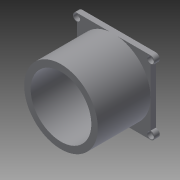
# Autodesk Inventor part: Nikon Mount
Saved by Autodesk Inventor 2013 (Build 170138000, 138)
## iProperties
Created: 2014-04-13
Part Number: Nikon Mount
Material: Generic
Document SubType Name: Modeling
Designer: spichelh
Density: 1 g/cm^3
Author: spichelh
Autodesk Inventor part; units mm, degrees
ref_plane "YZ Plane" through (0, 0, 0) normal (1, 0, 0) x (0, 1, 0)
ref_plane "XZ Plane" through (0, 0, 0) normal (0, 1, 0) x (-1, 0, 0)
ref_plane "XY Plane" through (0, 0, 0) normal (0, 0, 1) x (1, 0, 0)
sketch "Sketch1" plane through (0, 0, 0) normal (0, 0, 1) x (1, 0, 0)
  line L0 (55.88, 55.53) -> (0, 55.53)
  circle A0 centre (0, 3) radius 1.5
  arc A1 (0, 6) -> (0, 0) centre (0, 3) ccw
  circle A2 centre (0, 52.53) radius 1.5
  arc A3 (0, 55.53) -> (0, 49.53) centre (0, 52.53) ccw
  line L1 (27.94, 5) -> (27.94, 55.53) construction
  circle A4 centre (55.88, 3) radius 1.5
  arc A5 (55.88, 0) -> (55.88, 6) centre (55.88, 3) ccw
  circle A6 centre (55.88, 52.53) radius 1.5
  arc A7 (55.88, 49.53) -> (55.88, 55.53) centre (55.88, 52.53) ccw
  line L2 (55.88, 6) -> (55.88, 49.53)
  line L3 (55.88, 55.53) -> (55.88, 55.53)
  line L4 (0, 55.53) -> (0, 55.53)
  line L5 (0, 49.53) -> (0, 6)
  line L6 (52.88, 53.53) -> (3, 53.53)
  line L7 (0, 0) -> (0, 6) construction
  line L8 (55.88, 0) -> (55.88, 6) construction
  line L9 (0, 0) -> (0, 0)
  line L10 (0, 0) -> (55.88, 0)
  line L11 (55.88, 0) -> (55.88, 0)
  line L12 (50.88, 56.34) -> (5, 56.34) construction
  line L13 (3, 3) -> (52.88, 3)
  line L14 (3, 53.53) -> (3, 3)
  line L15 (52.88, 3) -> (52.88, 53.53)
  dimension "d0" = 55.88
  dimension "d2" = 3
  dimension "d3" = 6
  dimension "d4" = 3
  dimension "d5" = 6
  dimension "d6" = 49.53
  dimension "d8" = 3
  dimension "d14" = 2
  dimension "d33" = 0.81
  dimension "d78" = 3
  dimension "d79" = 3
  dimension "d214" = 0
  dimension "d215" = 3
  dimension "d216" = 0
  constraints: 32 end point, 9 parallel, 8 centre point, 8 point on circle, 5 coincident, 4 symmetric about line, 3 midpoint, 2 perpendicular, 1 collinear, 1 point on line, 4 other
  measures "d0" distance of L7.start L8.start
  measures "d2" diameter of A0
  measures "d3" diameter of A1
  measures "d4" diameter of A2
  measures "d5" diameter of A3
  measures "d6" distance of A0.centre A2.centre
  measures "d8" distance of A0.centre L7.start
  measures "d14" distance between parallel lines of L0 L6
  measures "d33" distance between parallel lines of L0 L12
  measures "d78" distance between parallel lines of L15 L2
  measures "d79" distance between parallel lines of L5 L14
  measures "d214" distance of L3.start L0.start
  measures "d215" distance between parallel lines of L10 L13
  measures "d216" distance of L9.end L7.start
extrude "Extrusion1" add sketch "Sketch1" along normal blind 4
sketch "Sketch14" plane through (0, 0, 4) normal (0, 0, 1) x (1, 0, 0)
  line L0 (3, 53.53) -> (52.88, 53.53)
  circle A0 centre (27.94, 27.765) radius 23
  line L1 (27.94, 53.53) -> (27.94, -2.5) construction
  line L2 (49.2166, 63.2696) -> (5.8766, 63.2721) construction
  line L3 (-23.2566, 6.5875) -> (78.3434, 6.5818) construction
  line L4 (-23.2534, 63.2737) -> (-23.2566, 6.5875) construction
  line L5 (78.3434, 6.5818) -> (78.3466, 63.268) construction
  line L6 (52.88, 53.53) -> (52.88, 3) projected
  line L7 (52.88, 3) -> (3, 3) projected
  line L8 (3, 3) -> (3, 53.53) projected
  line L9 (3, 3) -> (3, 53.53)
  line L10 (52.88, 53.53) -> (52.88, 3)
  line L11 (52.88, 3) -> (3, 3)
  point P0 (52.88, -2.5)
  dimension "d96" = 46
  constraints: 10 end point, 3 collinear, 1 centre point, 1 horizontal, 1 midpoint, 1 point on line
  measures "d96" diameter of A0
extrude "Extrusion14" add sketch "Sketch14" against normal blind 4
sketch "Sketch15" plane through (0, 0, 4) normal (0, 0, 1) x (1, 0, 0)
  circle A0 centre (27.94, 27.765) radius 23 projected
  line L0 (0, 49.53) -> (0, 6) projected
  circle A1 centre (27.94, 27.765) radius 27.94
  circle A2 centre (27.94, 27.765) radius 23
  dimension "d102" = 55.88
  dimension "d103" = 46
  constraints: 2 centre point, 2 coincident, 1 concentric, 1 tangent
  measures "d102" diameter of A1
  measures "d103" diameter of A0
extrude "Extrusion15" add sketch "Sketch15" along normal blind 40
sketch "Sketch17" plane through (0, 0, 0) normal (0, 0, -1) x (-1, 0, 0)
  circle A0 centre (-27.94, 27.765) radius 23 construction
  line L0 (-37.34, 35.815) -> (-18.54, 35.815)
  line L1 (-17.54, 34.815) -> (-17.54, 20.715)
  line L2 (-18.54, 19.715) -> (-37.34, 19.715)
  line L3 (-38.34, 20.715) -> (-38.34, 34.815)
  line L4 (-17.54, 35.815) -> (-38.34, 19.715) construction
  line L5 (-17.54, 19.715) -> (-38.34, 35.815) construction
  circle A1 centre (-27.94, 27.765) radius 23
  arc A2 (-37.34, 35.815) -> (-38.34, 34.815) centre (-37.34, 34.815) ccw
  arc A3 (-38.34, 20.715) -> (-37.34, 19.715) centre (-37.34, 20.715) ccw
  arc A4 (-18.54, 19.715) -> (-17.54, 20.715) centre (-18.54, 20.715) ccw
  arc A5 (-17.54, 34.815) -> (-18.54, 35.815) centre (-18.54, 34.815) ccw
  point P0 (0, 0)
  dimension "d111" = 20.8
  dimension "d112" = 16.1
  dimension "d115" = 1
  constraints: 12 end point, 8 point on circle, 8 point on line, 8 tangent, 5 centre point, 4 equal radius, 2 midpoint, 2 parallel, 1 coincident, 1 horizontal, 1 perpendicular
  measures "d111" distance of L5.start L4.end
  measures "d112" distance of L4.start L5.start
  measures "d115" radius of A2
extrude "Extrusion17" add sketch "Sketch17" against normal blind 11
sketch "Sketch18" plane through (27.94, 27.765, 11) normal (0, 0, 1) x (1, 0, 0)
  line L0 (10.4, 7.05) -> (10.4, -7.05) projected
  line L1 (9.4, -8.05) -> (-9.4, -8.05) projected
  line L2 (-10.4, -7.05) -> (-10.4, 7.05) projected
  line L3 (-9.4, 8.05) -> (9.4, 8.05) projected
  arc A0 (10.4, 7.05) -> (9.4, 8.05) centre (9.4, 7.05) ccw projected
  arc A1 (9.4, -8.05) -> (10.4, -7.05) centre (9.4, -7.05) ccw projected
  arc A2 (-10.4, -7.05) -> (-9.4, -8.05) centre (-9.4, -7.05) ccw projected
  arc A3 (-9.4, 8.05) -> (-10.4, 7.05) centre (-9.4, 7.05) ccw projected
  line L4 (9.4, 9.05) -> (-9.4, 9.05)
  arc A4 (-9.4, 9.05) -> (-11.4, 7.05) centre (-9.4, 7.05) ccw
  line L5 (-11.4, 7.05) -> (-11.4, -7.05)
  arc A5 (-11.4, -7.05) -> (-9.4, -9.05) centre (-9.4, -7.05) ccw
  line L6 (-9.4, -9.05) -> (9.4, -9.05)
  arc A6 (9.4, -9.05) -> (11.4, -7.05) centre (9.4, -7.05) ccw
  line L7 (11.4, -7.05) -> (11.4, 7.05)
  arc A7 (11.4, 7.05) -> (9.4, 9.05) centre (9.4, 7.05) ccw
  point P0 (10.4, 8.05)
  point P1 (10.4, -8.05)
  point P2 (-10.4, -8.05)
  point P3 (-10.4, 8.05)
  point P4 (-27.94, -27.765)
  dimension "d116" = 1
  constraints: 8 end point, 8 point on circle, 4 centre point, 7 other
  measures "d116" distance between parallel lines of L4 L3
extrude "Extrusion18" cut sketch "Sketch18" against normal blind 8
sketch "Sketch19" plane through (27.94, 27.765, 11) normal (0, 0, 1) x (1, 0, 0)
  arc A0 (-9.4, 9.05) -> (-11.4, 7.05) centre (-9.4, 7.05) ccw projected
  line L0 (-9.4, 9.05) -> (9.4, 9.05) projected
  arc A1 (11.4, 7.05) -> (9.4, 9.05) centre (9.4, 7.05) ccw projected
  line L1 (11.4, 7.05) -> (11.4, -7.05) projected
  arc A2 (9.4, -9.05) -> (11.4, -7.05) centre (9.4, -7.05) ccw projected
  line L2 (9.4, -9.05) -> (-9.4, -9.05) projected
  arc A3 (-11.4, -7.05) -> (-9.4, -9.05) centre (-9.4, -7.05) ccw projected
  line L3 (-11.4, -7.05) -> (-11.4, 7.05) projected
  line L4 (9.4, 10.05) -> (-9.4, 10.05)
  arc A4 (-9.4, 10.05) -> (-12.4, 7.05) centre (-9.4, 7.05) ccw
  line L5 (-12.4, 7.05) -> (-12.4, -7.05)
  arc A5 (-12.4, -7.05) -> (-9.4, -10.05) centre (-9.4, -7.05) ccw
  line L6 (-9.4, -10.05) -> (9.4, -10.05)
  arc A6 (9.4, -10.05) -> (12.4, -7.05) centre (9.4, -7.05) ccw
  line L7 (12.4, -7.05) -> (12.4, 7.05)
  arc A7 (12.4, 7.05) -> (9.4, 10.05) centre (9.4, 7.05) ccw
  point P0 (-27.94, -27.765)
  dimension "d119" = 1
  constraints: 8 end point, 8 point on circle, 4 centre point, 7 other
  measures "d119" distance between parallel lines of L0 L4
extrude "Extrusion19" cut sketch "Sketch19" against normal blind 7
sketch "Sketch20" plane through (27.94, 27.765, 11) normal (0, 0, 1) x (1, 0, 0)
  arc A0 (-9.4, 10.05) -> (-12.4, 7.05) centre (-9.4, 7.05) ccw projected
  line L0 (-9.4, 10.05) -> (9.4, 10.05) projected
  arc A1 (12.4, 7.05) -> (9.4, 10.05) centre (9.4, 7.05) ccw projected
  line L1 (12.4, 7.05) -> (12.4, -7.05) projected
  arc A2 (9.4, -10.05) -> (12.4, -7.05) centre (9.4, -7.05) ccw projected
  line L2 (9.4, -10.05) -> (-9.4, -10.05) projected
  arc A3 (-12.4, -7.05) -> (-9.4, -10.05) centre (-9.4, -7.05) ccw projected
  line L3 (-12.4, -7.05) -> (-12.4, 7.05) projected
  line L4 (9.4, 11.05) -> (-9.4, 11.05)
  arc A4 (-9.4, 11.05) -> (-13.4, 7.05) centre (-9.4, 7.05) ccw
  line L5 (-13.4, 7.05) -> (-13.4, -7.05)
  arc A5 (-13.4, -7.05) -> (-9.4, -11.05) centre (-9.4, -7.05) ccw
  line L6 (-9.4, -11.05) -> (9.4, -11.05)
  arc A6 (9.4, -11.05) -> (13.4, -7.05) centre (9.4, -7.05) ccw
  line L7 (13.4, -7.05) -> (13.4, 7.05)
  arc A7 (13.4, 7.05) -> (9.4, 11.05) centre (9.4, 7.05) ccw
  point P0 (-27.94, -27.765)
  dimension "d122" = 1
  constraints: 8 end point, 8 point on circle, 4 centre point, 7 other
  measures "d122" distance between parallel lines of L4 L0
extrude "Extrusion20" cut sketch "Sketch20" against normal blind 6
sketch "Sketch21" plane through (27.94, 27.765, 11) normal (0, 0, 1) x (1, 0, 0)
  arc A0 (-9.4, 11.05) -> (-13.4, 7.05) centre (-9.4, 7.05) ccw projected
  line L0 (-9.4, 11.05) -> (9.4, 11.05) projected
  arc A1 (13.4, 7.05) -> (9.4, 11.05) centre (9.4, 7.05) ccw projected
  line L1 (13.4, 7.05) -> (13.4, -7.05) projected
  arc A2 (9.4, -11.05) -> (13.4, -7.05) centre (9.4, -7.05) ccw projected
  line L2 (9.4, -11.05) -> (-9.4, -11.05) projected
  arc A3 (-13.4, -7.05) -> (-9.4, -11.05) centre (-9.4, -7.05) ccw projected
  line L3 (-13.4, -7.05) -> (-13.4, 7.05) projected
  line L4 (9.4, 12.05) -> (-9.4, 12.05)
  arc A4 (-9.4, 12.05) -> (-14.4, 7.05) centre (-9.4, 7.05) ccw
  line L5 (-14.4, 7.05) -> (-14.4, -7.05)
  arc A5 (-14.4, -7.05) -> (-9.4, -12.05) centre (-9.4, -7.05) ccw
  line L6 (-9.4, -12.05) -> (9.4, -12.05)
  arc A6 (9.4, -12.05) -> (14.4, -7.05) centre (9.4, -7.05) ccw
  line L7 (14.4, -7.05) -> (14.4, 7.05)
  arc A7 (14.4, 7.05) -> (9.4, 12.05) centre (9.4, 7.05) ccw
  point P0 (-27.94, -27.765)
  dimension "d125" = 1
  constraints: 8 end point, 8 point on circle, 4 centre point, 7 other
  measures "d125" distance between parallel lines of L0 L4
extrude "Extrusion21" cut sketch "Sketch21" against normal blind 5
sketch "Sketch22" plane through (27.94, 27.765, 11) normal (0, 0, 1) x (1, 0, 0)
  arc A0 (-9.4, 12.05) -> (-14.4, 7.05) centre (-9.4, 7.05) ccw projected
  line L0 (-9.4, 12.05) -> (9.4, 12.05) projected
  arc A1 (14.4, 7.05) -> (9.4, 12.05) centre (9.4, 7.05) ccw projected
  line L1 (14.4, 7.05) -> (14.4, -7.05) projected
  arc A2 (9.4, -12.05) -> (14.4, -7.05) centre (9.4, -7.05) ccw projected
  line L2 (9.4, -12.05) -> (-9.4, -12.05) projected
  arc A3 (-14.4, -7.05) -> (-9.4, -12.05) centre (-9.4, -7.05) ccw projected
  line L3 (-14.4, -7.05) -> (-14.4, 7.05) projected
  line L4 (9.4, 13.05) -> (-9.4, 13.05)
  arc A4 (-9.4, 13.05) -> (-15.4, 7.05) centre (-9.4, 7.05) ccw
  line L5 (-15.4, 7.05) -> (-15.4, -7.05)
  arc A5 (-15.4, -7.05) -> (-9.4, -13.05) centre (-9.4, -7.05) ccw
  line L6 (-9.4, -13.05) -> (9.4, -13.05)
  arc A6 (9.4, -13.05) -> (15.4, -7.05) centre (9.4, -7.05) ccw
  line L7 (15.4, -7.05) -> (15.4, 7.05)
  arc A7 (15.4, 7.05) -> (9.4, 13.05) centre (9.4, 7.05) ccw
  point P0 (-27.94, -27.765)
  dimension "d128" = 1
  constraints: 8 end point, 8 point on circle, 4 centre point, 7 other
  measures "d128" distance between parallel lines of L0 L4
extrude "Extrusion22" cut sketch "Sketch22" against normal blind 4
sketch "Sketch23" plane through (27.94, 27.765, 11) normal (0, 0, 1) x (1, 0, 0)
  arc A0 (-9.4, 13.05) -> (-15.4, 7.05) centre (-9.4, 7.05) ccw projected
  line L0 (-9.4, 13.05) -> (9.4, 13.05) projected
  arc A1 (15.4, 7.05) -> (9.4, 13.05) centre (9.4, 7.05) ccw projected
  line L1 (15.4, 7.05) -> (15.4, -7.05) projected
  arc A2 (9.4, -13.05) -> (15.4, -7.05) centre (9.4, -7.05) ccw projected
  line L2 (9.4, -13.05) -> (-9.4, -13.05) projected
  arc A3 (-15.4, -7.05) -> (-9.4, -13.05) centre (-9.4, -7.05) ccw projected
  line L3 (-15.4, -7.05) -> (-15.4, 7.05) projected
  line L4 (9.4, 14.05) -> (-9.4, 14.05)
  arc A4 (-9.4, 14.05) -> (-16.4, 7.05) centre (-9.4, 7.05) ccw
  line L5 (-16.4, 7.05) -> (-16.4, -7.05)
  arc A5 (-16.4, -7.05) -> (-9.4, -14.05) centre (-9.4, -7.05) ccw
  line L6 (-9.4, -14.05) -> (9.4, -14.05)
  arc A6 (9.4, -14.05) -> (16.4, -7.05) centre (9.4, -7.05) ccw
  line L7 (16.4, -7.05) -> (16.4, 7.05)
  arc A7 (16.4, 7.05) -> (9.4, 14.05) centre (9.4, 7.05) ccw
  point P0 (-27.94, -27.765)
  dimension "d131" = 1
  constraints: 8 end point, 8 point on circle, 4 centre point, 7 other
  measures "d131" distance between parallel lines of L0 L4
extrude "Extrusion23" cut sketch "Sketch23" against normal blind 3
sketch "Sketch24" plane through (27.94, 27.765, 11) normal (0, 0, 1) x (1, 0, 0)
  arc A0 (-9.4, 14.05) -> (-16.4, 7.05) centre (-9.4, 7.05) ccw projected
  line L0 (-9.4, 14.05) -> (9.4, 14.05) projected
  arc A1 (16.4, 7.05) -> (9.4, 14.05) centre (9.4, 7.05) ccw projected
  line L1 (16.4, 7.05) -> (16.4, -7.05) projected
  arc A2 (9.4, -14.05) -> (16.4, -7.05) centre (9.4, -7.05) ccw projected
  line L2 (9.4, -14.05) -> (-9.4, -14.05) projected
  arc A3 (-16.4, -7.05) -> (-9.4, -14.05) centre (-9.4, -7.05) ccw projected
  line L3 (-16.4, -7.05) -> (-16.4, 7.05) projected
  line L4 (9.4, 15.05) -> (-9.4, 15.05)
  arc A4 (-9.4, 15.05) -> (-17.4, 7.05) centre (-9.4, 7.05) ccw
  line L5 (-17.4, 7.05) -> (-17.4, -7.05)
  arc A5 (-17.4, -7.05) -> (-9.4, -15.05) centre (-9.4, -7.05) ccw
  line L6 (-9.4, -15.05) -> (9.4, -15.05)
  arc A6 (9.4, -15.05) -> (17.4, -7.05) centre (9.4, -7.05) ccw
  line L7 (17.4, -7.05) -> (17.4, 7.05)
  arc A7 (17.4, 7.05) -> (9.4, 15.05) centre (9.4, 7.05) ccw
  point P0 (-27.94, -27.765)
  dimension "d134" = 1
  constraints: 8 end point, 8 point on circle, 4 centre point, 7 other
  measures "d134" distance between parallel lines of L0 L4
extrude "Extrusion24" cut sketch "Sketch24" against normal blind 2
sketch "Sketch25" plane through (27.94, 27.765, 11) normal (0, 0, 1) x (1, 0, 0)
  arc A0 (-9.4, 15.05) -> (-17.4, 7.05) centre (-9.4, 7.05) ccw projected
  line L0 (-9.4, 15.05) -> (9.4, 15.05) projected
  arc A1 (17.4, 7.05) -> (9.4, 15.05) centre (9.4, 7.05) ccw projected
  line L1 (17.4, 7.05) -> (17.4, -7.05) projected
  arc A2 (9.4, -15.05) -> (17.4, -7.05) centre (9.4, -7.05) ccw projected
  line L2 (9.4, -15.05) -> (-9.4, -15.05) projected
  arc A3 (-17.4, -7.05) -> (-9.4, -15.05) centre (-9.4, -7.05) ccw projected
  line L3 (-17.4, -7.05) -> (-17.4, 7.05) projected
  line L4 (9.4, 16.05) -> (-9.4, 16.05)
  arc A4 (-9.4, 16.05) -> (-18.4, 7.05) centre (-9.4, 7.05) ccw
  line L5 (-18.4, 7.05) -> (-18.4, -7.05)
  arc A5 (-18.4, -7.05) -> (-9.4, -16.05) centre (-9.4, -7.05) ccw
  line L6 (-9.4, -16.05) -> (9.4, -16.05)
  arc A6 (9.4, -16.05) -> (18.4, -7.05) centre (9.4, -7.05) ccw
  line L7 (18.4, -7.05) -> (18.4, 7.05)
  arc A7 (18.4, 7.05) -> (9.4, 16.05) centre (9.4, 7.05) ccw
  point P0 (-27.94, -27.765)
  dimension "d137" = 1
  constraints: 8 end point, 8 point on circle, 4 centre point, 7 other
  measures "d137" distance between parallel lines of L0 L4
extrude "Extrusion25" cut sketch "Sketch25" against normal blind 1
sketch "Sketch31" plane through (0, 0, 4) normal (0, 0, 1) x (1, 0, 0)
  circle A0 centre (0, 3) radius 1.5 projected
  circle A1 centre (55.88, 3) radius 1.5 projected
  circle A2 centre (0, 3) radius 2.5
  circle A3 centre (55.88, 3) radius 2.5
  arc A4 (55.88, 27.765) -> (31.0622, 55.53) centre (27.94, 27.765) ccw projected
  line L0 (55.88, 27.765) -> (55.88, 49.53) projected
  arc A5 (55.88, 49.53) -> (55.88, 55.53) centre (55.88, 52.53) ccw projected
  line L1 (55.88, 55.53) -> (31.0622, 55.53) projected
  arc A6 (0, 55.53) -> (0, 49.53) centre (0, 52.53) ccw projected
  line L2 (0, 49.53) -> (0, 27.765) projected
  circle A7 centre (55.88, 52.53) radius 1.5 projected
  circle A8 centre (0, 52.53) radius 1.5 projected
  circle A9 centre (0, 52.53) radius 2.5
  circle A10 centre (55.88, 52.53) radius 2.5
  line L3 (0, 27.765) -> (0, 6) projected
  arc A11 (0, 6) -> (0, 0) centre (0, 3) ccw projected
  line L4 (0, 0) -> (24.8178, 0) projected
  arc A12 (55.88, 0) -> (55.88, 6) centre (55.88, 3) ccw projected
  line L5 (55.88, 6) -> (55.88, 27.765) projected
  arc A13 (24.8178, 55.53) -> (0, 27.765) centre (27.94, 27.765) ccw projected
  arc A14 (0, 27.765) -> (24.8178, 0) centre (27.94, 27.765) ccw projected
  arc A15 (31.0622, 0) -> (55.88, 27.765) centre (27.94, 27.765) ccw projected
  line L6 (31.0622, 0) -> (55.88, 0) projected
  line L7 (24.8178, 55.53) -> (0, 55.53) projected
  dimension "d172" = 5
  dimension "d174" = 5
  dimension "d175" = 5
  dimension "d176" = 5
  constraints: 4 centre point, 4 coincident
  measures "d172" diameter of A2
  measures "d174" diameter of A3
  measures "d175" diameter of A9
  measures "d176" diameter of A10
extrude "Extrusion31" cut sketch "Sketch31" against normal blind 3 contours A2 | A3 | A9 | A10
sketch "Sketch39" plane through (0, 0, 0) normal (0, 0, -1) x (-1, 0, 0)
  arc A0 (-38.34, 20.715) -> (-37.34, 19.715) centre (-37.34, 20.715) ccw projected
  line L0 (-38.34, 20.715) -> (-38.34, 34.815) projected
  arc A1 (-37.34, 35.815) -> (-38.34, 34.815) centre (-37.34, 34.815) ccw projected
  line L1 (-37.34, 35.815) -> (-18.54, 35.815) projected
  arc A2 (-17.54, 34.815) -> (-18.54, 35.815) centre (-18.54, 34.815) ccw projected
  line L2 (-17.54, 34.815) -> (-17.54, 20.715) projected
  arc A3 (-18.54, 19.715) -> (-17.54, 20.715) centre (-18.54, 20.715) ccw projected
  line L3 (-18.54, 19.715) -> (-37.34, 19.715) projected
  line L4 (-40.44, 40.265) -> (-15.44, 40.265)
  line L5 (-15.44, 40.265) -> (-15.44, 15.265)
  line L6 (-15.44, 15.265) -> (-40.44, 15.265)
  line L7 (-40.44, 15.265) -> (-40.44, 40.265)
  line L8 (-15.44, 40.265) -> (-40.44, 15.265) construction
  line L9 (-40.44, 40.265) -> (-15.44, 15.265) construction
  line L10 (-18.54, 20.715) -> (-37.34, 34.815) construction
  line L11 (-37.34, 20.715) -> (-18.54, 34.815) construction
  point P0 (-27.94, 27.765)
  dimension "d217" = 25
  dimension "d219" = 25
  constraints: 16 end point, 3 midpoint, 2 parallel, 1 horizontal, 1 perpendicular
  measures "d217" distance of L4.start L4.end
  measures "d219" distance of L4.end L5.end
extrude "Extrusion38" cut sketch "Sketch39" against normal blind 1.6
sketch "Sketch40" plane through (0, 0, 1.6) normal (0, 0, -1) x (-1, 0, 0)
  line L0 (-37.34, 19.715) -> (-18.54, 19.715) projected
  arc A0 (-38.34, 20.715) -> (-37.34, 19.715) centre (-37.34, 20.715) ccw projected
  line L1 (-38.34, 34.815) -> (-38.34, 20.715) projected
  arc A1 (-37.34, 35.815) -> (-38.34, 34.815) centre (-37.34, 34.815) ccw projected
  line L2 (-18.54, 35.815) -> (-37.34, 35.815) projected
  arc A2 (-17.54, 34.815) -> (-18.54, 35.815) centre (-18.54, 34.815) ccw projected
  line L3 (-17.54, 20.715) -> (-17.54, 34.815) projected
  arc A3 (-18.54, 19.715) -> (-17.54, 20.715) centre (-18.54, 20.715) ccw projected
  line L4 (-40.44, 40.265) -> (-15.44, 40.265) projected
  line L5 (-40.44, 15.265) -> (-40.44, 40.265) projected
  line L6 (-15.44, 15.265) -> (-40.44, 15.265) projected
  line L7 (-15.44, 40.265) -> (-15.44, 15.265) projected
  line L8 (-15.44, 40.265) -> (-40.44, 15.265) construction
  line L9 (-15.44, 15.265) -> (-40.44, 40.265) construction
  point P0 (0, 0)
  point P1 (-27.94, 27.765)
  constraints: 4 end point, 1 midpoint, 1 perpendicular
body "Solid1"
